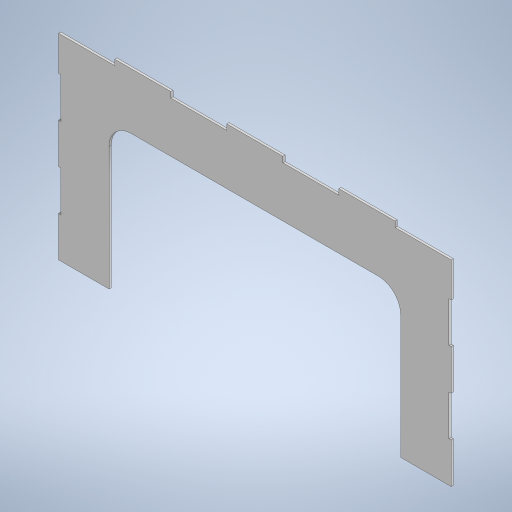
# Autodesk Inventor part: back
Saved by Autodesk Inventor 2023 (Build 270158000, 158)
## iProperties
Created: 2023-04-26
Part Number: back
Material: Generic
Document SubType Name: Modeling
Designer: Unnar
Density: 1 g/cm^3
Appearance: Default
Author: Unnar
Autodesk Inventor part; units mm, degrees
ref_plane "YZ Plane" through (0, 0, 0) normal (1, 0, 0) x (0, 1, 0)
ref_plane "XZ Plane" through (0, 0, 0) normal (0, 1, 0) x (-1, 0, 0)
ref_plane "XY Plane" through (0, 0, 0) normal (0, 0, 1) x (1, 0, 0)
sketch "Sketch1" plane through (0, 0, 0) normal (0, 0, 1) x (1, 0, 0)
  line L0 (-179.7163, 90.3709) -> (170.2837, 90.3709)
  line L1 (170.2837, 90.3709) -> (170.2837, -89.6291)
  line L2 (-179.7163, -89.6291) -> (-179.7163, 90.3709)
  line L3 (125.2837, -89.6291) -> (125.2837, 20.3709)
  line L4 (105.2837, 40.3709) -> (-114.7163, 40.3709)
  line L5 (-134.7163, 20.3709) -> (-134.7163, -89.6291)
  line L6 (170.2837, -89.6291) -> (125.2837, -89.6291)
  line L7 (-134.7163, -89.6291) -> (-179.7163, -89.6291)
  arc A0 (-114.7163, 40.3709) -> (-134.7163, 20.3709) centre (-114.7163, 20.3709) ccw
  arc A1 (125.2837, 20.3709) -> (105.2837, 40.3709) centre (105.2837, 20.3709) ccw
  point P0 (0, 0)
  dimension "d0" = 350
  dimension "d1" = 180
  dimension "d2" = 45
  dimension "d3" = 45
  dimension "d4" = 50
  dimension "d5" = 20
  constraints: 16 end point, 4 parallel, 4 point on circle, 4 tangent, 2 centre point, 1 equal radius, 1 horizontal, 1 perpendicular
  measures "d0" distance of L0.start L0.end
  measures "d1" distance of L0.end L1.end
  measures "d2" distance of L5.end L2.start
  measures "d3" distance of L1.end L3.start
  measures "d4" distance between parallel lines of L4 L0
  measures "d5" radius of A0
extrude "Extrusion1" add sketch "Sketch1" along normal blind 2
sketch "Sketch2" plane through (0, 0, 2) normal (0, 0, 1) x (1, 0, 0)
  line L0 (170.2837, 90.3709) -> (-179.7163, 90.3709) projected
  line L1 (-179.7163, 90.3709) -> (-129.7163, 90.3709)
  line L2 (-129.7163, 90.3709) -> (-129.7163, 85.3709)
  line L3 (-129.7163, 85.3709) -> (-179.7163, 85.3709)
  line L4 (-179.7163, 85.3709) -> (-179.7163, 90.3709)
  line L5 (-79.7163, 90.3709) -> (-29.7163, 90.3709)
  line L6 (-29.7163, 90.3709) -> (-29.7163, 85.3709)
  line L7 (-29.7163, 85.3709) -> (-79.7163, 85.3709)
  line L8 (-79.7163, 85.3709) -> (-79.7163, 90.3709)
  line L9 (20.2837, 90.3709) -> (70.2837, 90.3709)
  line L10 (70.2837, 90.3709) -> (70.2837, 85.3709)
  line L11 (70.2837, 85.3709) -> (20.2837, 85.3709)
  line L12 (20.2837, 85.3709) -> (20.2837, 90.3709)
  line L13 (170.2837, 90.3709) -> (120.2837, 90.3709)
  line L14 (120.2837, 90.3709) -> (120.2837, 85.3709)
  line L15 (120.2837, 85.3709) -> (170.2837, 85.3709)
  line L16 (170.2837, 85.3709) -> (170.2837, 90.3709)
  point P0 (0, 0)
  dimension "d8" = 50
  dimension "d9" = 50
  dimension "d10" = 50
  dimension "d11" = 50
  dimension "d12" = 50
  dimension "d13" = 50
  dimension "d14" = 50
  dimension "d15" = 5
  constraints: 32 end point, 8 parallel, 5 point on line, 4 horizontal, 4 perpendicular
  measures "d8" distance of L2.end L3.end
  measures "d9" distance of L6.end L7.end
  measures "d10" distance of L10.end L11.end
  measures "d11" distance of L14.end L15.end
  measures "d12" distance between parallel lines of L10 L14
  measures "d13" distance between parallel lines of L8 L2
  measures "d14" distance between parallel lines of L12 L6
  measures "d15" distance of L1.end L2.end
extrude "Extrusion2" cut sketch "Sketch2" against normal blind 2
sketch "Sketch3" plane through (0, 0, 2) normal (0, 0, 1) x (1, 0, 0)
  line L0 (-179.7163, 85.3709) -> (-179.7163, -89.6291) projected
  line L1 (-179.7163, -53.6291) -> (-177.7163, -53.6291)
  line L2 (-177.7163, -53.6291) -> (-177.7163, -17.6291)
  line L3 (-177.7163, -17.6291) -> (-179.7163, -17.6291)
  line L4 (-179.7163, -17.6291) -> (-179.7163, -53.6291)
  line L5 (-179.7163, 18.3709) -> (-177.7163, 18.3709)
  line L6 (-177.7163, 18.3709) -> (-177.7163, 54.3709)
  line L7 (-177.7163, 54.3709) -> (-179.7163, 54.3709)
  line L8 (-179.7163, 54.3709) -> (-179.7163, 18.3709)
  line L9 (170.2837, -89.6291) -> (170.2837, 85.3709) projected
  line L10 (170.2837, -53.6291) -> (168.2837, -53.6291)
  line L11 (168.2837, -53.6291) -> (168.2837, -17.6291)
  line L12 (168.2837, -17.6291) -> (170.2837, -17.6291)
  line L13 (170.2837, -17.6291) -> (170.2837, -53.6291)
  line L14 (170.2837, 18.3709) -> (168.2837, 18.3709)
  line L15 (168.2837, 18.3709) -> (168.2837, 54.3709)
  line L16 (168.2837, 54.3709) -> (170.2837, 54.3709)
  line L17 (170.2837, 54.3709) -> (170.2837, 18.3709)
  line L18 (-179.7163, -89.6291) -> (-134.7163, -89.6291) projected
  line L19 (125.2837, -89.6291) -> (170.2837, -89.6291) projected
  point P0 (-177.7163, -35.6291)
  point P1 (-178.7163, -53.6291)
  point P2 (-178.7163, -17.6291)
  point P3 (-178.7163, 18.3709)
  point P4 (169.2837, -17.6291)
  point P5 (169.2837, 18.3709)
  point P6 (169.2837, -53.6291)
  dimension "d28" = 36
  dimension "d29" = 2
  dimension "d30" = 2
  dimension "d31" = 36
  dimension "d32" = 36
  dimension "d33" = 36
  dimension "d34" = 2
  dimension "d35" = 36
  dimension "d36" = 36
  dimension "d37" = 36
  dimension "d38" = 36
  constraints: 32 end point, 9 point on line, 8 parallel, 7 midpoint, 4 horizontal, 4 perpendicular
  measures "d28" distance of L5.end L6.end
  measures "d29" distance from line of L0 point (-177.716, -35.629)
  measures "d30" distance between parallel lines of L0 L6
  measures "d31" distance of L1.end L2.end
  measures "d32" distance from line of L18 point (-178.716, -53.629)
  measures "d33" distance of point (-178.716, -17.629) point (-178.716, 18.371)
  measures "d34" distance between parallel lines of L9 L15
  measures "d35" distance of L10.end L11.end
  measures "d36" distance of L14.end L15.end
  measures "d37" distance of point (169.284, -17.629) point (169.284, 18.371)
  measures "d38" distance from line of L19 point (169.284, -53.629)
extrude "Extrusion3" cut sketch "Sketch3" against normal blind 2
body "Solid1"
